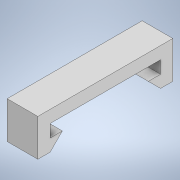
# Autodesk Inventor part: Тестовая крышка
Saved by Autodesk Inventor 2020 (Build 240168000, 168)
## iProperties
Created: 2021-04-26
Part Number: Тестовая крышка
Material: Типовые
Document SubType Name: Modeling
Designer: Антон
Density: 1 g/cm^3
Appearance: По умолчанию
Author: Антон
Autodesk Inventor part; units mm, degrees
ref_plane "YZ Plane" through (0, 0, 0) normal (1, 0, 0) x (0, 1, 0)
ref_plane "XZ Plane" through (0, 0, 0) normal (0, 1, 0) x (-1, 0, 0)
ref_plane "XY Plane" through (0, 0, 0) normal (0, 0, 1) x (1, 0, 0)
sketch "Эскиз1" plane through (0, 0, 0) normal (0, 1, 0) x (-1, 0, 0)
  line L0 (0, 0) -> (5, 0)
  line L1 (5, 0) -> (5, -9)
  line L2 (5, -9) -> (0, -9)
  line L3 (0, -9) -> (0, 0)
  dimension "d0" = 5
  dimension "d1" = 9
  constraints: 8 end point, 2 parallel, 1 horizontal, 1 perpendicular
  measures "d0" distance of L1.end L2.end
  measures "d1" distance of L0.end L1.end
extrude "Выдавливание1" add sketch "Эскиз1" along normal blind 2
sketch "Эскиз2" plane through (-5, 0, -9) normal (-1, 0, 0) x (0, 0, 1)
  line L0 (9, 2) -> (0, 2) projected
  line L1 (9, 2) -> (11, 2)
  line L2 (11, 2) -> (11, -4.05)
  line L3 (11, -4.05) -> (9, -4.05)
  line L4 (9, -4.05) -> (9, 2)
  line L5 (9, -4.05) -> (7, -4.05)
  line L6 (7, -4.05) -> (7, -2.05)
  line L7 (7, -2.05) -> (9, -2.05)
  line L8 (9, -2.05) -> (9, -4.05)
  line L9 (7, -2.05) -> (9, -4.05)
  point P0 (9, 0)
  dimension "d4" = 2
  dimension "d5" = 6.05
  dimension "d6" = 2
  dimension "d7" = 2
  constraints: 18 end point, 4 parallel, 2 horizontal, 2 perpendicular
  measures "d4" distance of L2.end L3.end
  measures "d5" distance between parallel lines of L3 L1
  measures "d6" distance of L6.end L7.end
  measures "d7" distance of L5.end L6.end
extrude "Выдавливание2" add sketch "Эскиз2" against normal blind 5 contours L1 L2 L3 L4 | L4 L9 L7
mirror "Зеркальное отражение1" about plane through (0, 0, -9) normal (0, 0, -1)
